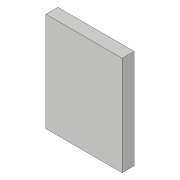
# Autodesk Inventor part: 328 Adafruit 2.5 Ah Lithium Battery
Saved by Autodesk Inventor 2018.3 (Build 223284000, 284)
## iProperties
Created: 2018-12-11
Part Number: 328 Adafruit 2.5 Ah Lithium Battery
Material: Generic
Document SubType Name: Modeling
Designer: tei06398
Mass: 25.6194 g
Surface Area: 83.1934 cm^2
Volume: 25.6194 cm^3
Density: 1 g/cm^3
Appearance: Default
Author: tei06398
Autodesk Inventor part; units mm, degrees
ref_plane "YZ Plane" through (0, 0, 0) normal (1, 0, 0) x (0, 1, 0)
ref_plane "XZ Plane" through (0, 0, 0) normal (0, 1, 0) x (-1, 0, 0)
ref_plane "XY Plane" through (0, 0, 0) normal (0, 0, 1) x (1, 0, 0)
sketch "Sketch1" plane through (0, 0, 0) normal (0, 0, 1) x (1, 0, 0)
  line L0 (0, 0) -> (50.038, 0)
  line L1 (50.038, 0) -> (50.038, 65.024)
  line L2 (50.038, 65.024) -> (0, 65.024)
  line L3 (0, 65.024) -> (0, 0)
  dimension "d0" = 50.038
  dimension "d1" = 65.024
  constraints: 8 end point, 2 parallel, 1 horizontal, 1 perpendicular
  measures "d0" distance of L2.end L1.end
  measures "d1" distance of L1.end L0.end
extrude "Extrusion1" add sketch "Sketch1" against normal blind 7.874
body "Solid1"
